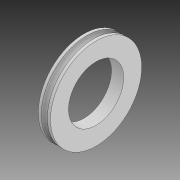
# Autodesk Inventor part: Cablecar_idlepulley
Saved by Autodesk Inventor 2020 (Build 240168000, 168)
## iProperties
Created: 2021-02-03
Part Number: Cablecar_idlepulley
Material: Generic
Document SubType Name: Modeling
Designer: DDeGo
Density: 1 g/cm^3
Appearance: Default
Author: DDeGo
Autodesk Inventor part; units mm, degrees
ref_plane "YZ Plane" through (0, 0, 0) normal (1, 0, 0) x (0, 1, 0)
ref_plane "XZ Plane" through (0, 0, 0) normal (0, 1, 0) x (-1, 0, 0)
ref_plane "XY Plane" through (0, 0, 0) normal (0, 0, 1) x (1, 0, 0)
sketch "Sketch1" plane through (0, 0, 0) normal (0, 0, 1) x (1, 0, 0)
  arc A0 (1, 0) -> (-1, 0) centre (0, 0) ccw
  line L0 (-2, 0) -> (-1, 0)
  line L1 (-1, 0) -> (1, 0) construction
  line L2 (1, 0) -> (2, 0)
  line L3 (2, 0) -> (2, 5.93)
  line L4 (2, 5.93) -> (-2, 5.93)
  line L5 (-2, 5.93) -> (-2, 0)
  line L6 (-2, 5.93) -> (-2, 15) construction
  line L7 (-2, 15) -> (2, 15) construction
  line L8 (2, 15) -> (2, 5.93) construction
  dimension "d0" = 4
  dimension "d1" = 1
  dimension "d2" = 9.07
  dimension "d3" = 15
  constraints: 18 end point, 5 perpendicular, 2 coincident, 2 point on circle, 2 point on line, 1 centre point, 1 collinear, 1 horizontal, 1 midpoint, 1 vertical
  measures "d0" distance between parallel lines of L3 L5
  measures "d1" radius of A0
  measures "d2" distance between parallel lines of L4 L7
  measures "d3" distance between parallel lines of L7 L2
revolve "Revolution1" add sketch "Sketch1" angle 360 about axis through (-2, 15, 0) along (1, 0, 0)
body "Solid1"
